Autodesk Fusion 360 part; units mm, degrees
note: some values were not read from the file. Chosen so that the rebuilt part matches the saved one: that a step has no effect.
(part 6 of 7)
  spline S243 degree 3 poles (23.9288, 79.9512) (23.18, 79.2024) (22.4312, 78.4536) (21.6597, 77.6822) knots 0 0 0 0 1 1 1 1
  spline S244 degree 3 poles (21.6597, 77.6822) (21.5445, 77.7398) (21.4293, 77.7974) (21.3106, 77.8567) knots 0 0 0 0 1 1 1 1
  spline S245 degree 3 poles (21.3106, 77.8567) (22.7527, 79.5314) (22.7527, 79.5314) (23.5797, 80.1258) knots 0 0 0 0 1 1 1 1
  spline S246 degree 3 poles (-14.8203, 67.384) (-14.7051, 67.3264) (-14.5899, 67.2688) (-14.4712, 67.2094) knots 0 0 0 0 1 1 1 1
  spline S247 degree 3 poles (-14.4712, 67.2094) (-15.0472, 66.6334) (-15.6232, 66.0574) (-16.2166, 65.464) knots 0 0 0 0 1 1 1 1
  spline S248 degree 3 poles (-16.2166, 65.464) (-16.3318, 65.5216) (-16.447, 65.5792) (-16.5657, 65.6385) knots 0 0 0 0 1 1 1 1
  spline S249 degree 3 poles (-16.5657, 65.6385) (-16.5081, 65.7537) (-16.4505, 65.8689) (-16.3912, 65.9876) knots 0 0 0 0 1 1 1 1
  spline S250 degree 3 poles (-16.3912, 65.9876) (-16.276, 65.9876) (-16.1608, 65.9876) (-16.0421, 65.9876) knots 0 0 0 0 1 1 1 1
  spline S251 degree 3 poles (-16.0421, 65.9876) (-16.0421, 66.1028) (-16.0421, 66.218) (-16.0421, 66.3367) knots 0 0 0 0 1 1 1 1
  spline S252 degree 3 poles (-16.0421, 66.3367) (-15.9269, 66.3367) (-15.8117, 66.3367) (-15.693, 66.3367) knots 0 0 0 0 1 1 1 1
  spline S253 degree 3 poles (-15.693, 66.3367) (-15.693, 66.4519) (-15.693, 66.5671) (-15.693, 66.6858) knots 0 0 0 0 1 1 1 1
  spline S254 degree 3 poles (-15.693, 66.6858) (-15.5778, 66.6858) (-15.4626, 66.6858) (-15.3439, 66.6858) knots 0 0 0 0 1 1 1 1
  spline S255 degree 3 poles (-15.3439, 66.6858) (-15.2863, 66.8586) (-15.2287, 67.0314) (-15.1694, 67.2094) knots 0 0 0 0 1 1 1 1
  spline S256 degree 3 poles (-15.1694, 67.2094) (-15.0542, 67.267) (-14.939, 67.3246) (-14.8203, 67.384) knots 0 0 0 0 1 1 1 1
  spline S257 degree 3 poles (-17.2639, 64.7658) (-17.0911, 64.6506) (-16.9183, 64.5354) (-16.7403, 64.4167) knots 0 0 0 0 1 1 1 1
  spline S258 degree 3 poles (-16.7403, 64.4167) (-16.9357, 64.2411) (-17.1323, 64.0668) (-17.3293, 63.8931) knots 0 0 0 0 1 1 1 1
  spline S259 degree 3 poles (-17.3293, 63.8931) (-17.4387, 63.7959) (-17.548, 63.6987) (-17.6607, 63.5985) knots 0 0 0 0 1 1 1 1
  spline S260 degree 3 poles (-17.6607, 63.5985) (-17.9621, 63.3694) (-17.9621, 63.3694) (-18.3112, 63.3694) knots 0 0 0 0 1 1 1 1
  spline S261 degree 3 poles (-18.3112, 63.3694) (-18.3112, 63.4846) (-18.3112, 63.5998) (-18.3112, 63.7185) knots 0 0 0 0 1 1 1 1
  spline S262 degree 3 poles (-18.3112, 63.7185) (-18.196, 63.7185) (-18.0808, 63.7185) (-17.9621, 63.7185) knots 0 0 0 0 1 1 1 1
  spline S263 degree 3 poles (-17.9621, 63.7185) (-17.9621, 63.8337) (-17.9621, 63.9489) (-17.9621, 64.0676) knots 0 0 0 0 1 1 1 1
  spline S264 degree 3 poles (-17.9621, 64.0676) (-17.8469, 64.0676) (-17.7317, 64.0676) (-17.613, 64.0676) knots 0 0 0 0 1 1 1 1
  spline S265 degree 3 poles (-17.613, 64.0676) (-17.4978, 64.298) (-17.3826, 64.5284) (-17.2639, 64.7658) knots 0 0 0 0 1 1 1 1
sketch "Sketch101" plane through (71.6406, 0, 0) normal (-1, 0, 0) x (0, -1, 0)
  line L0 (57.3648, 64.7338) -> (57.3648, 39.3343)
  line L1 (54.3648, 39.3343) -> (54.3648, 64.7338)
  line L2 (57.3648, 39.3343) -> (54.3648, 39.3343)
  line L3 (54.3648, 39.3343) -> (54.3648, 19.7124)
  line L4 (54.3648, 19.7124) -> (57.3648, 19.7124)
  line L5 (57.3648, 19.7124) -> (57.3648, 39.3343)
  line L6 (57.3648, 39.3343) -> (54.3648, 39.3343)
  line L7 (54.3648, 39.3343) -> (54.3648, 59.6271)
  line L8 (54.3648, 59.6271) -> (57.3648, 59.6271)
  line L9 (57.3648, 59.6271) -> (57.3648, 39.3343)
  constraint horizontal L2
  constraint vertical L3
  constraint horizontal L4
  constraint vertical L5
  constraint coincident L0.end L2.start
  constraint horizontal L6
  constraint vertical L7
  constraint horizontal L8
  constraint vertical L9
  constraint coincident L1 L7.end
extrude "Extrude4" cut sketch "Sketch101" along normal blind 172 and the other way blind 2 bodies 2 in component "Component"
sketch "Sketch102" plane through (0, -58.3648, 0) normal (0, -1, 0) x (1, 0, 0)
  line L0 (76.6406, 106.1458) -> (-103.3594, 106.1458)
  line L1 (-103.3594, 106.1458) -> (-103.3594, 16.8343)
  line L2 (-103.3594, 16.8343) -> (-98.3594, 16.8343)
  line L3 (-98.3594, 16.8343) -> (-98.3594, 39.3343)
  line L4 (-98.3594, 39.3343) -> (-23.3594, 39.3343)
  line L5 (-23.3594, 39.3343) -> (-23.3594, 75)
  line L6 (-23.3594, 75) -> (-3.3594, 75)
  line L7 (-3.3594, 75) -> (-3.3594, 39.3343)
  line L8 (-3.3594, 39.3343) -> (71.6406, 39.3343)
  line L9 (71.6406, 39.3343) -> (71.6406, 16.8343)
  line L10 (71.6406, 16.8343) -> (76.6406, 16.8343)
  line L11 (76.6406, 16.8343) -> (76.6406, 106.1458)
sketch "Sketch103" plane through (0, -58.3648, 0) normal (0, -1, 0) x (1, 0, 0)
  line L0 (-3.3594, 39.3343) -> (-3.3594, 86.8343)
  line L1 (-23.3594, 75) -> (-3.3594, 75)
  line L2 (-23.3594, 39.3343) -> (-23.3594, 75)
  line L3 (-98.3594, 39.3343) -> (-23.3594, 39.3343)
  line L4 (-3.3594, 39.3343) -> (71.6406, 39.3343)
  line L5 (71.6406, 39.3343) -> (71.6406, 16.8343)
  line L6 (76.6406, 16.8343) -> (76.6406, 111.8343)
  line L7 (71.6406, 19.7124) -> (-98.3594, 19.7124)
  line L8 (-98.3594, 16.8343) -> (-98.3594, 39.3343)
  line L9 (-103.3594, 111.8343) -> (-103.3594, 16.8343)
  line L10 (74.0853, 19.7124) -> (-99.6129, 19.7124)
  line L11 (-99.6129, 19.7124) -> (-99.6129, 81.8546)
  line L12 (-99.6129, 81.8546) -> (74.0853, 81.8546)
  line L13 (74.0853, 81.8546) -> (74.0853, 19.7124)
  constraint horizontal L10
  constraint vertical L11
  constraint horizontal L12
  constraint vertical L13
extrude "Extrude32" add sketch "Sketch103" along normal blind 2.5 separate body makes body 3
move_body "Move18" bodies 3 to x (1, 0, 0) y (0, 1, 0) z (0, 0, 1) at (0, -47, 0)
move_body "Move19" bodies 3 to x (1, 0, 0) y (0, 1, 0) z (0, 0, 1) at (0, 50, 0)
sketch "Sketch104" plane through (0, -57.8648, 0) normal (0, -1, 0) x (1, 0, 0)
  line L0 (74.0853, 81.8546) -> (-99.6129, 81.8546)
  line L1 (-99.6129, 81.8546) -> (-99.6129, 19.7124)
  line L2 (-99.6129, 19.7124) -> (74.0853, 19.7124)
  line L3 (74.0853, 19.7124) -> (74.0853, 81.8546)
  line L4 (-8, 43) -> (-19, 43)
  line L5 (-19, 43) -> (-19, 49)
  line L6 (-19, 49) -> (-8, 49)
  line L7 (-8, 49) -> (-8, 43)
  constraint horizontal L4
  constraint vertical L5
  constraint horizontal L6
  constraint vertical L7
extrude "Extrude33" cut sketch "Sketch104" against normal blind 11 contours L4 L5 L6 L7 bodies 3
move_body "Move20" bodies 3 to x (1, 0, 0) y (0, 1, 0) z (0, 0, 1) at (0, -60, 0)
sketch "Sketch105" plane through (0, 0, 0) normal (0, 0, 1) x (1, 0, 0)
sketch "Sketch106" plane through (0, 0, 0) normal (0, 0, 1) x (1, 0, 0)
  line L0 (10, -170) -> (-1, -170)
  line L1 (-1, -170) -> (-1, -162.5)
  line L2 (-1, -162.5) -> (10, -162.5)
  line L3 (10, -162.5) -> (10, -170)
  line L4 (-1, -162.5) -> (2, -162.5)
  line L5 (2, -162.5) -> (2, -158)
  line L6 (2, -158) -> (-1, -158)
  line L7 (-1, -158) -> (-1, -162.5)
  line L8 (10, -162.5) -> (7, -162.5)
  line L9 (7, -162.5) -> (7, -158)
  line L10 (7, -158) -> (10, -158)
  line L11 (10, -158) -> (10, -162.5)
  line L12 (-1, -158) -> (-1, -159.85)
  line L13 (-1, -159.85) -> (-2.25, -159.85)
  line L14 (-2.25, -159.85) -> (-1, -158)
  line L15 (10, -158) -> (10, -159.85)
  line L16 (10, -159.85) -> (11.25, -159.85)
  line L17 (11.25, -159.85) -> (10, -158)
  line L18 (10, -170) -> (11.25, -170)
  line L19 (11.25, -170) -> (11.25, -162.5)
  line L20 (11.25, -162.5) -> (10, -162.5)
  line L21 (10, -162.5) -> (10, -170)
  line L22 (-1, -170) -> (-2.25, -170)
  line L23 (-2.25, -170) -> (-2.25, -162.5)
  line L24 (-2.25, -162.5) -> (-1, -162.5)
  line L25 (-1, -162.5) -> (-1, -170)
  dimension "d167" = 11
  dimension "d168" = 7.5
  dimension "d169" = 4.5
  dimension "d170" = 1.85
  dimension "d171" = 1.25
  dimension "d172" = 1.85
  dimension "d173" = 1.25
  dimension "d174" = 1.25
  dimension "d175" = 1.25
  constraint horizontal L0
  constraint vertical L1
  constraint horizontal L2
  constraint vertical L3
  constraint horizontal L4
  constraint vertical L5
  constraint horizontal L6
  constraint vertical L7
  constraint horizontal L8
  constraint vertical L9
  constraint horizontal L10
  constraint vertical L11
  constraint coincident L7 L12.end
  constraint perpendicular L12 L13
  constraint coincident L11 L15.end
  constraint perpendicular L11 L16
  constraint horizontal L18
  constraint vertical L19
  constraint horizontal L20
  constraint vertical L21
  constraint horizontal L22
  constraint vertical L23
  constraint horizontal L24
  constraint vertical L25
  measures "d167" distance of L0.start L0.end
  measures "d168" distance of L0.start L2.end
  measures "d169" distance of L1.end L6.end
  measures "d170" distance of L6.end L12.end
  measures "d171" distance of L12.end L13.end
  measures "d172" distance of L10.end L15.end
  measures "d173" distance of L15.end L16.end
  measures "d174" distance of L0.start L18.end
  measures "d175" distance of L0.end L22.end
extrude "Extrude34" add sketch "Sketch106" along normal blind 6 separate body makes body 4
fillet "Fillet4" radius 6 tangency weight 1.3685 1 edges at (4.5, -170, 6) on bodies 4
sketch "Sketch59" plane through (-89.5415, 0, 0) normal (-1, 0, 0) x (0, -1, 0)
sketch "Sketch60" plane through (0, 0, 0) normal (1, 0, 0) x (0, 1, 0)
sketch "Sketch107" plane through (0, 66.6352, 0) normal (0, 1, 0) x (-1, 0, 0)
  line L0 (103.3594, 140.242) -> (-76.6406, 140.242)
  line L1 (-76.6406, 140.242) -> (-76.6406, 16.8343)
  line L2 (-76.6406, 16.8343) -> (103.3594, 16.8343)
  line L3 (103.3594, 16.8343) -> (103.3594, 140.242)
  spline S0 degree 3 poles (-45.7064, 96.8261) (-45.5481, 96.8681) (-45.3897, 96.9101) (-45.2266, 96.9534) knots 0 0 0 0 1 1 1 1
  spline S1 degree 3 poles (-45.2266, 96.9534) (-42.4795, 97.6788) (-39.7486, 98.2533) (-36.9248, 98.5683) knots 0 0 0 0 1 1 1 1
  spline S2 degree 3 poles (-36.9248, 98.5683) (-36.7802, 98.5846) (-36.7802, 98.5846) (-36.6326, 98.6012) knots 0 0 0 0 1 1 1 1
  spline S3 degree 3 poles (-36.6326, 98.6012) (-25.791, 99.8038) (-14.8744, 98.8757) (-3.0729, 96.8273) knots 0 0 0 0 1 1 1 1
  spline S4 degree 3 poles (-3.0729, 96.8273) (8.3921, 94.7476) (19.8407, 95.0185) (31.1023, 98.0497) knots 0 0 0 0 1 1 1 1
  spline S5 degree 3 poles (31.1023, 98.0497) (31.2954, 98.1015) (31.2954, 98.1015) (31.4923, 98.1544) knots 0 0 0 0 1 1 1 1
  spline S6 degree 3 poles (31.4923, 98.1544) (33.7602, 98.766) (35.989, 99.441) (38.1951, 100.2513) knots 0 0 0 0 1 1 1 1
  spline S7 degree 3 poles (38.1951, 100.2513) (38.2806, 100.2826) (38.3662, 100.3138) (38.4543, 100.3461) knots 0 0 0 0 1 1 1 1
  spline S8 degree 3 poles (38.4543, 100.3461) (48.019, 103.8522) (56.949, 108.978) (65.0365, 115.1519) knots 0 0 0 0 1 1 1 1
  spline S9 degree 3 poles (65.0365, 115.1519) (65.1117, 115.2093) (65.1868, 115.2666) (65.2643, 115.3258) knots 0 0 0 0 1 1 1 1
  spline S10 degree 3 poles (65.2643, 115.3258) (69.065, 118.2344) (72.9424, 121.3668) (76.1266, 124.9512) knots 0 0 0 0 1 1 1 1
  spline S11 degree 3 poles (76.1266, 124.9512) (76.5375, 125.3995) (76.5375, 125.3995) (76.9194, 125.4556) knots 0 0 0 0 1 1 1 1
  spline S12 degree 3 poles (76.9194, 125.4556) (77.0345, 125.4372) (77.0345, 125.4372) (77.152, 125.4185) knots 0 0 0 0 1 1 1 1
  spline S13 degree 3 poles (77.152, 125.4185) (77.4126, 125.0218) (77.4195, 124.9501) (77.3533, 124.4429) knots 0 0 0 0 1 1 1 1
  spline S14 degree 3 poles (77.3533, 124.4429) (77.3089, 124.2369) (77.2625, 124.0312) (77.2147, 123.8259) knots 0 0 0 0 1 1 1 1
  spline S15 degree 3 poles (77.2147, 123.8259) (77.1901, 123.7141) (77.1655, 123.6022) (77.1402, 123.4869) knots 0 0 0 0 1 1 1 1
  spline S16 degree 3 poles (77.1402, 123.4869) (77.0586, 123.1177) (76.9746, 122.749) (76.8906, 122.3803) knots 0 0 0 0 1 1 1 1
  spline S17 degree 3 poles (76.8906, 122.3803) (76.8333, 122.1227) (76.7762, 121.865) (76.7192, 121.6073) knots 0 0 0 0 1 1 1 1
  spline S18 degree 3 poles (76.7192, 121.6073) (76.6019, 121.0775) (76.4837, 120.5479) (76.3648, 120.0184) knots 0 0 0 0 1 1 1 1
  spline S19 degree 3 poles (76.3648, 120.0184) (76.2043, 119.3015) (76.0477, 118.5839) (75.8931, 117.8657) knots 0 0 0 0 1 1 1 1
  spline S20 degree 3 poles (75.8931, 117.8657) (75.8697, 117.7573) (75.8464, 117.6488) (75.8223, 117.5371) knots 0 0 0 0 1 1 1 1
  spline S21 degree 3 poles (75.8223, 117.5371) (75.7761, 117.3223) (75.7299, 117.1075) (75.6837, 116.8927) knots 0 0 0 0 1 1 1 1
  spline S22 degree 3 poles (75.6837, 116.8927) (75.4001, 115.5741) (75.1139, 114.2561) (74.8196, 112.9399) knots 0 0 0 0 1 1 1 1
  spline S23 degree 3 poles (74.8196, 112.9399) (74.7781, 112.7534) (74.7365, 112.5669) (74.695, 112.3805) knots 0 0 0 0 1 1 1 1
  spline S24 degree 3 poles (74.695, 112.3805) (74.6179, 112.035) (74.5401, 111.6897) (74.4619, 111.3445) knots 0 0 0 0 1 1 1 1
  spline S25 degree 3 poles (74.4619, 111.3445) (74.4282, 111.1936) (74.3945, 111.0428) (74.3598, 110.8874) knots 0 0 0 0 1 1 1 1
  spline S26 degree 3 poles (74.3598, 110.8874) (74.3301, 110.7558) (74.3004, 110.6243) (74.2697, 110.4887) knots 0 0 0 0 1 1 1 1
  spline S27 degree 3 poles (74.2697, 110.4887) (74.1941, 110.1853) (74.1941, 110.1853) (74.2842, 109.9213) knots 0 0 0 0 1 1 1 1
  spline S28 degree 3 poles (74.2842, 109.9213) (76.0956, 110.302) (77.8875, 110.7306) (79.6733, 111.2173) knots 0 0 0 0 1 1 1 1
  spline S29 degree 3 poles (79.6733, 111.2173) (80.0659, 111.3243) (80.4588, 111.4304) (80.8516, 111.5364) knots 0 0 0 0 1 1 1 1
  spline S30 degree 3 poles (80.8516, 111.5364) (81.6816, 111.7603) (82.5112, 111.9853) (83.3409, 112.2104) knots 0 0 0 0 1 1 1 1
  spline S31 degree 3 poles (83.3409, 112.2104) (84.3124, 112.474) (85.284, 112.7371) (86.2558, 112.9991) knots 0 0 0 0 1 1 1 1
  spline S32 degree 3 poles (86.2558, 112.9991) (86.6428, 113.1037) (87.0296, 113.2091) (87.4163, 113.3145) knots 0 0 0 0 1 1 1 1
  spline S33 degree 3 poles (87.4163, 113.3145) (87.6511, 113.3779) (87.8859, 113.4412) (88.1207, 113.5046) knots 0 0 0 0 1 1 1 1
  spline S34 degree 3 poles (88.1207, 113.5046) (88.228, 113.5341) (88.3354, 113.5635) (88.446, 113.5939) knots 0 0 0 0 1 1 1 1
  spline S35 degree 3 poles (88.446, 113.5939) (89.1834, 113.7916) (89.1834, 113.7916) (89.5079, 113.7252) knots 0 0 0 0 1 1 1 1
  spline S36 degree 3 poles (89.5079, 113.7252) (89.5844, 113.1789) (89.5219, 112.9091) (89.2263, 112.4463) knots 0 0 0 0 1 1 1 1
  spline S37 degree 3 poles (89.2263, 112.4463) (89.156, 112.3347) (89.0857, 112.2231) (89.0134, 112.1081) knots 0 0 0 0 1 1 1 1
  spline S38 degree 3 poles (89.0134, 112.1081) (88.9387, 111.9931) (88.864, 111.8782) (88.787, 111.7598) knots 0 0 0 0 1 1 1 1
  spline S39 degree 3 poles (88.787, 111.7598) (88.6798, 111.5902) (88.6798, 111.5902) (88.5704, 111.4173) knots 0 0 0 0 1 1 1 1
  spline S40 degree 3 poles (88.5704, 111.4173) (87.8976, 110.3582) (87.1937, 109.32) (86.483, 108.2861) knots 0 0 0 0 1 1 1 1
  spline S41 degree 3 poles (86.483, 108.2861) (86.049, 107.6537) (85.6171, 107.0201) (85.188, 106.3844) knots 0 0 0 0 1 1 1 1
  spline S42 degree 3 poles (85.188, 106.3844) (84.1912, 104.9075) (83.192, 103.4375) (82.1157, 102.017) knots 0 0 0 0 1 1 1 1
  spline S43 degree 3 poles (82.1157, 102.017) (81.6377, 101.3842) (81.1782, 100.7395) (80.7206, 100.0918) knots 0 0 0 0 1 1 1 1
  spline S44 degree 3 poles (80.7206, 100.0918) (80.0586, 99.1578) (79.3691, 98.2516) (78.6566, 97.3557) knots 0 0 0 0 1 1 1 1
  spline S45 degree 3 poles (78.6566, 97.3557) (78.2349, 96.8249) (77.8215, 96.288) (77.4084, 95.7505) knots 0 0 0 0 1 1 1 1
  spline S46 degree 3 poles (77.4084, 95.7505) (76.5588, 94.6451) (75.7018, 93.5492) (74.8053, 92.4814) knots 0 0 0 0 1 1 1 1
  spline S47 degree 3 poles (74.8053, 92.4814) (74.5969, 92.2324) (74.39, 91.9821) (74.1832, 91.7317) knots 0 0 0 0 1 1 1 1
  spline S48 degree 3 poles (74.1832, 91.7317) (67.0705, 83.1524) (59.1895, 75.0046) (40.5169, 63.8451) knots 0 0 0 0 1 1 1 1
  spline S49 degree 3 poles (40.5169, 63.8451) (40.3871, 63.7934) (40.2573, 63.7418) (40.1236, 63.6886) knots 0 0 0 0 1 1 1 1
  spline S50 degree 3 poles (40.1236, 63.6886) (28.4595, 59.163) (14.8221, 57.7208) (-16.1582, 57.4264) knots 0 0 0 0 1 1 1 1
  spline S51 degree 3 poles (-16.1582, 57.4264) (-32.9463, 58.0691) (-32.9463, 58.0691) (-50.0558, 56.645) knots 0 0 0 0 1 1 1 1
  spline S52 degree 3 poles (-50.0558, 56.645) (-50.1821, 56.6269) (-50.3084, 56.6088) (-50.4385, 56.5901) knots 0 0 0 0 1 1 1 1
  spline S53 degree 3 poles (-50.4385, 56.5901) (-54.3089, 56.0263) (-58.132, 54.9004) (-61.7438, 53.4135) knots 0 0 0 0 1 1 1 1
  spline S54 degree 3 poles (-61.7438, 53.4135) (-62.1127, 53.2747) (-62.4824, 53.1713) (-62.8645, 53.0753) knots 0 0 0 0 1 1 1 1
  spline S55 degree 3 poles (-62.8645, 53.0753) (-62.2573, 46.7418) (-61.3762, 40.5103) (-59.846, 34.3289) knots 0 0 0 0 1 1 1 1
  spline S56 degree 3 poles (-59.846, 34.3289) (-59.778, 34.0527) (-59.71, 33.7766) (-59.642, 33.5004) knots 0 0 0 0 1 1 1 1
  spline S57 degree 3 poles (-59.642, 33.5004) (-59.4776, 32.8323) (-59.3124, 32.1643) (-59.1472, 31.4964) knots 0 0 0 0 1 1 1 1
  spline S58 degree 3 poles (-59.1472, 31.4964) (-60.7154, 31.0762) (-62.2835, 30.656) (-63.8992, 30.2231) knots 0 0 0 0 1 1 1 1
  spline S59 degree 3 poles (-63.8992, 30.2231) (-67.1692, 41.0011) (-67.0232, 53.7045) (-63.94, 78.6656) knots 0 0 0 0 1 1 1 1
  spline S60 degree 3 poles (-63.94, 78.6656) (-63.9131, 78.8142) (-63.8861, 78.9628) (-63.8583, 79.1159) knots 0 0 0 0 1 1 1 1
  spline S61 degree 3 poles (-63.8583, 79.1159) (-63.665, 80.175) (-63.4644, 81.2325) (-63.2592, 82.2893) knots 0 0 0 0 1 1 1 1
  spline S62 degree 3 poles (-63.2592, 82.2893) (-63.2291, 82.4451) (-63.1989, 82.6008) (-63.1679, 82.7613) knots 0 0 0 0 1 1 1 1
  spline S63 degree 3 poles (-63.1679, 82.7613) (-61.8055, 89.7543) (-61.8055, 89.7543) (-61.1055, 90.6265) knots 0 0 0 0 1 1 1 1
  spline S64 degree 3 poles (-61.1055, 90.6265) (-60.7716, 90.8303) (-60.4678, 90.9184) (-60.0835, 90.9864) knots 0 0 0 0 1 1 1 1
  spline S65 degree 3 poles (-60.0835, 90.9864) (-59.7353, 90.7854) (-59.6641, 90.6676) (-59.4917, 90.3191) knots 0 0 0 0 1 1 1 1
  spline S66 degree 3 poles (-59.4917, 90.3191) (-59.4098, 90.3895) (-59.3279, 90.4599) (-59.2435, 90.5324) knots 0 0 0 0 1 1 1 1
  spline S67 degree 3 poles (-59.2435, 90.5324) (-55.3519, 93.7416) (-50.5292, 95.5611) (-45.7064, 96.8261) knots 0 0 0 0 1 1 1 1
  spline S68 degree 3 poles (-48.2512, 87.4119) (-47.2839, 87.3215) (-46.6105, 86.7927) (-45.9714, 86.0957) knots 0 0 0 0 1 1 1 1
  spline S69 degree 3 poles (-45.9714, 86.0957) (-45.6421, 85.688) (-45.3536, 85.2668) (-45.0791, 84.8206) knots 0 0 0 0 1 1 1 1
  spline S70 degree 3 poles (-45.0791, 84.8206) (-45.024, 84.7314) (-44.9689, 84.6422) (-44.9121, 84.5503) knots 0 0 0 0 1 1 1 1
  spline S71 degree 3 poles (-44.9121, 84.5503) (-44.1771, 83.2187) (-43.8013, 81.5801) (-43.8059, 80.0686) knots 0 0 0 0 1 1 1 1
  spline S72 degree 3 poles (-43.8059, 80.0686) (-43.7534, 79.8533) (-43.697, 79.6389) (-43.6338, 79.4265) knots 0 0 0 0 1 1 1 1
  spline S73 degree 3 poles (-43.6338, 79.4265) (-42.0204, 79.1867) (-40.4101, 78.9482) (-38.7854, 78.7985) knots 0 0 0 0 1 1 1 1
  spline S74 degree 3 poles (-38.7854, 78.7985) (-38.7949, 78.8939) (-38.8045, 78.9892) (-38.8144, 79.0875) knots 0 0 0 0 1 1 1 1
  spline S75 degree 3 poles (-38.8144, 79.0875) (-38.8299, 79.4995) (-38.7836, 79.8578) (-38.714, 80.264) knots 0 0 0 0 1 1 1 1
  spline S76 degree 3 poles (-38.714, 80.264) (-38.688, 80.417) (-38.6619, 80.57) (-38.635, 80.7276) knots 0 0 0 0 1 1 1 1
  spline S77 degree 3 poles (-38.635, 80.7276) (-38.6063, 80.8899) (-38.5775, 81.0522) (-38.5479, 81.2194) knots 0 0 0 0 1 1 1 1
  spline S78 degree 3 poles (-38.5479, 81.2194) (-38.5186, 81.3862) (-38.4893, 81.553) (-38.4591, 81.7249) knots 0 0 0 0 1 1 1 1
  spline S79 degree 3 poles (-38.4591, 81.7249) (-38.276, 82.7484) (-38.0824, 83.769) (-37.86, 84.7848) knots 0 0 0 0 1 1 1 1
  spline S80 degree 3 poles (-37.86, 84.7848) (-37.837, 84.8937) (-37.8139, 85.0025) (-37.7901, 85.1147) knots 0 0 0 0 1 1 1 1
  spline S81 degree 3 poles (-37.7901, 85.1147) (-37.5744, 86.0609) (-37.2674, 87.0489) (-36.4835, 87.6744) knots 0 0 0 0 1 1 1 1
  spline S82 degree 3 poles (-36.4835, 87.6744) (-35.8146, 87.9652) (-35.173, 88.1221) (-34.4492, 88.013) knots 0 0 0 0 1 1 1 1
  spline S83 degree 3 poles (-34.4492, 88.013) (-33.7177, 87.6026) (-33.1504, 87.1937) (-32.9061, 86.3596) knots 0 0 0 0 1 1 1 1
  spline S84 degree 3 poles (-32.9061, 86.3596) (-32.6181, 85.1833) (-32.6635, 83.9595) (-32.6534, 82.7558) knots 0 0 0 0 1 1 1 1
  spline S85 degree 3 poles (-32.6534, 82.7558) (-32.6518, 82.6241) (-32.6501, 82.4924) (-32.6484, 82.3567) knots 0 0 0 0 1 1 1 1
  spline S86 degree 3 poles (-32.6484, 82.3567) (-32.6146, 79.6527) (-32.6761, 76.9545) (-32.7882, 74.253) knots 0 0 0 0 1 1 1 1
  spline S87 degree 3 poles (-32.7882, 74.253) (-32.8012, 73.9352) (-32.8133, 73.6174) (-32.8251, 73.2995) knots 0 0 0 0 1 1 1 1
  spline S88 degree 3 poles (-32.8251, 73.2995) (-32.8438, 72.8023) (-32.8641, 72.3051) (-32.886, 71.808) knots 0 0 0 0 1 1 1 1
  spline S89 degree 3 poles (-32.886, 71.808) (-32.8975, 71.5439) (-32.9079, 71.2798) (-32.9184, 71.0157) knots 0 0 0 0 1 1 1 1
  spline S90 degree 3 poles (-32.9184, 71.0157) (-33.0049, 69.2409) (-33.1993, 67.4218) (-34.4428, 66.0593) knots 0 0 0 0 1 1 1 1
  spline S91 degree 3 poles (-34.4428, 66.0593) (-35.0109, 65.5526) (-35.6375, 65.3103) (-36.3967, 65.2604) knots 0 0 0 0 1 1 1 1
  spline S92 degree 3 poles (-36.3967, 65.2604) (-36.9978, 65.4856) (-37.2892, 65.7801) (-37.6399, 66.3038) knots 0 0 0 0 1 1 1 1
  spline S93 degree 3 poles (-37.6399, 66.3038) (-38.0544, 67.3349) (-38.0845, 68.4101) (-38.111, 69.507) knots 0 0 0 0 1 1 1 1
  spline S94 degree 3 poles (-38.111, 69.507) (-38.1217, 69.831) (-38.1327, 70.155) (-38.144, 70.479) knots 0 0 0 0 1 1 1 1
  spline S95 degree 3 poles (-38.144, 70.479) (-38.1492, 70.6346) (-38.1543, 70.7903) (-38.1597, 70.9506) knots 0 0 0 0 1 1 1 1
  spline S96 degree 3 poles (-38.1597, 70.9506) (-38.1938, 71.8188) (-38.2651, 72.6835) (-38.3423, 73.5488) knots 0 0 0 0 1 1 1 1
  spline S97 degree 3 poles (-38.3423, 73.5488) (-38.416, 73.549) (-38.4896, 73.5492) (-38.5655, 73.5494) knots 0 0 0 0 1 1 1 1
  spline S98 degree 3 poles (-38.5655, 73.5494) (-39.7226, 73.5671) (-40.8652, 73.7004) (-42.0137, 73.8297) knots 0 0 0 0 1 1 1 1
  spline S99 degree 3 poles (-42.0137, 73.8297) (-42.2191, 73.8524) (-42.4245, 73.8751) (-42.6299, 73.8977) knots 0 0 0 0 1 1 1 1
  spline S100 degree 3 poles (-42.6299, 73.8977) (-43.128, 73.9527) (-43.6261, 74.0083) (-44.1241, 74.0643) knots 0 0 0 0 1 1 1 1
  spline S101 degree 3 poles (-44.1241, 74.0643) (-44.1289, 73.9442) (-44.1337, 73.8241) (-44.1387, 73.7003) knots 0 0 0 0 1 1 1 1
  spline S102 degree 3 poles (-44.1387, 73.7003) (-44.1936, 72.9724) (-44.3564, 72.2721) (-44.512, 71.5599) knots 0 0 0 0 1 1 1 1
  spline S103 degree 3 poles (-44.512, 71.5599) (-44.5686, 71.2988) (-44.6228, 71.0371) (-44.677, 70.7755) knots 0 0 0 0 1 1 1 1
  spline S104 degree 3 poles (-44.677, 70.7755) (-44.9743, 69.4058) (-45.3183, 68.0168) (-46.3334, 66.9941) knots 0 0 0 0 1 1 1 1
  spline S105 degree 3 poles (-46.3334, 66.9941) (-46.432, 66.8923) (-46.5305, 66.7905) (-46.632, 66.6856) knots 0 0 0 0 1 1 1 1
  spline S106 degree 3 poles (-46.632, 66.6856) (-47.2185, 66.1416) (-47.8826, 65.9502) (-48.6622, 65.8281) knots 0 0 0 0 1 1 1 1
  spline S107 degree 3 poles (-48.6622, 65.8281) (-49.2058, 65.9712) (-49.5103, 66.1644) (-49.8365, 66.6147) knots 0 0 0 0 1 1 1 1
  spline S108 degree 3 poles (-49.8365, 66.6147) (-50.4305, 68.1882) (-50.5246, 69.623) (-50.3988, 71.2818) knots 0 0 0 0 1 1 1 1
  spline S109 degree 3 poles (-50.3988, 71.2818) (-50.1218, 75.1545) (-50.1421, 78.9743) (-50.4328, 82.8449) knots 0 0 0 0 1 1 1 1
  spline S110 degree 3 poles (-50.4328, 82.8449) (-50.6339, 85.6223) (-50.6339, 85.6223) (-49.977, 86.4677) knots 0 0 0 0 1 1 1 1
  spline S111 degree 3 poles (-49.977, 86.4677) (-49.9171, 86.5476) (-49.8573, 86.6276) (-49.7956, 86.7099) knots 0 0 0 0 1 1 1 1
  spline S112 degree 3 poles (-49.7956, 86.7099) (-49.3755, 87.2034) (-48.8822, 87.3316) (-48.2512, 87.4119) knots 0 0 0 0 1 1 1 1
  spline S113 degree 3 poles (-60.0835, 90.9864) (-59.9223, 90.8933) (-59.9223, 90.8933) (-59.7578, 90.7984) knots 0 0 0 0 1 1 1 1
  spline S114 degree 3 poles (-59.7578, 90.7984) (-59.6284, 90.1547) (-59.6564, 89.6237) (-59.7823, 88.9835) knots 0 0 0 0 1 1 1 1
  spline S115 degree 3 poles (-59.7823, 88.9835) (-59.8155, 88.8087) (-59.8487, 88.6338) (-59.8818, 88.4589) knots 0 0 0 0 1 1 1 1
  spline S116 degree 3 poles (-59.8818, 88.4589) (-59.8999, 88.3664) (-59.918, 88.2739) (-59.9366, 88.1786) knots 0 0 0 0 1 1 1 1
  spline S117 degree 3 poles (-59.9366, 88.1786) (-61.1903, 81.7212) (-61.9509, 75.1546) (-62.5143, 68.604) knots 0 0 0 0 1 1 1 1
  spline S118 degree 3 poles (-62.5143, 68.604) (-62.5403, 68.3024) (-62.5667, 68.001) (-62.5932, 67.6995) knots 0 0 0 0 1 1 1 1
  spline S119 degree 3 poles (-62.5932, 67.6995) (-63.012, 62.906) (-63.2982, 58.0622) (-62.8373, 53.2629) knots 0 0 0 0 1 1 1 1
  spline S120 degree 3 poles (-62.8373, 53.2629) (-62.7985, 52.8482) (-62.7622, 52.4335) (-62.7269, 52.0185) knots 0 0 0 0 1 1 1 1
  spline S121 degree 3 poles (-62.7269, 52.0185) (-62.2171, 46.0375) (-61.2886, 40.1566) (-59.846, 34.3289) knots 0 0 0 0 1 1 1 1
  spline S122 degree 3 poles (-59.846, 34.3289) (-59.778, 34.0527) (-59.71, 33.7766) (-59.642, 33.5004) knots 0 0 0 0 1 1 1 1
  spline S123 degree 3 poles (-59.642, 33.5004) (-59.4776, 32.8323) (-59.3124, 32.1643) (-59.1472, 31.4964) knots 0 0 0 0 1 1 1 1
  spline S124 degree 3 poles (-59.1472, 31.4964) (-60.7154, 31.0762) (-62.2835, 30.656) (-63.8992, 30.2231) knots 0 0 0 0 1 1 1 1
  spline S125 degree 3 poles (-63.8992, 30.2231) (-67.1692, 41.0011) (-67.0232, 53.7045) (-63.94, 78.6656) knots 0 0 0 0 1 1 1 1
  spline S126 degree 3 poles (-63.94, 78.6656) (-63.9131, 78.8142) (-63.8861, 78.9628) (-63.8583, 79.1159) knots 0 0 0 0 1 1 1 1
  spline S127 degree 3 poles (-63.8583, 79.1159) (-63.665, 80.175) (-63.4644, 81.2325) (-63.2592, 82.2893) knots 0 0 0 0 1 1 1 1
  spline S128 degree 3 poles (-63.2592, 82.2893) (-63.2291, 82.4451) (-63.1989, 82.6008) (-63.1679, 82.7613) knots 0 0 0 0 1 1 1 1
  spline S129 degree 3 poles (-63.1679, 82.7613) (-61.8055, 89.7543) (-61.8055, 89.7543) (-61.1055, 90.6265) knots 0 0 0 0 1 1 1 1
  spline S130 degree 3 poles (-61.1055, 90.6265) (-60.7716, 90.8303) (-60.4678, 90.9184) (-60.0835, 90.9864) knots 0 0 0 0 1 1 1 1
  spline S131 degree 3 poles (-21.8651, 89.1136) (-20.6908, 88.715) (-19.8867, 87.8368) (-19.3239, 86.7576) knots 0 0 0 0 1 1 1 1
  spline S132 degree 3 poles (-19.3239, 86.7576) (-16.9734, 81.8605) (-16.4757, 75.9409) (-16.3625, 70.5683) knots 0 0 0 0 1 1 1 1
  spline S133 degree 3 poles (-16.3625, 70.5683) (-16.3598, 70.4405) (-16.3571, 70.3127) (-16.3543, 70.181) knots 0 0 0 0 1 1 1 1
  spline S134 degree 3 poles (-16.3543, 70.181) (-16.3393, 68.545) (-16.5087, 67.1547) (-17.5603, 65.8318) knots 0 0 0 0 1 1 1 1
  spline S135 degree 3 poles (-17.5603, 65.8318) (-18.072, 65.3272) (-18.6716, 65.0325) (-19.3953, 64.9981) knots 0 0 0 0 1 1 1 1
  spline S136 degree 3 poles (-19.3953, 64.9981) (-19.9203, 65.1264) (-20.2664, 65.3255) (-20.5696, 65.7847) knots 0 0 0 0 1 1 1 1
  spline S137 degree 3 poles (-20.5696, 65.7847) (-20.8221, 66.5469) (-20.8732, 67.1817) (-20.8262, 67.9786) knots 0 0 0 0 1 1 1 1
  spline S138 degree 3 poles (-20.8262, 67.9786) (-20.8212, 68.0853) (-20.8162, 68.192) (-20.811, 68.302) knots 0 0 0 0 1 1 1 1
  spline S139 degree 3 poles (-20.811, 68.302) (-20.7948, 68.6391) (-20.7764, 68.9761) (-20.758, 69.3131) knots 0 0 0 0 1 1 1 1
  spline S140 degree 3 poles (-20.758, 69.3131) (-20.7465, 69.5432) (-20.7352, 69.7734) (-20.7241, 70.0035) knots 0 0 0 0 1 1 1 1
  spline S141 degree 3 poles (-20.7241, 70.0035) (-20.6966, 70.5643) (-20.6672, 71.125) (-20.6366, 71.6857) knots 0 0 0 0 1 1 1 1
  spline S142 degree 3 poles (-20.6366, 71.6857) (-20.7837, 71.6554) (-20.9308, 71.625) (-21.0824, 71.5937) knots 0 0 0 0 1 1 1 1
  spline S143 degree 3 poles (-21.0824, 71.5937) (-23.0119, 71.1956) (-23.0119, 71.1956) (-23.9734, 71.0067) knots 0 0 0 0 1 1 1 1
  spline S144 degree 3 poles (-23.9734, 71.0067) (-24.2164, 70.9589) (-24.2164, 70.9589) (-24.4642, 70.9102) knots 0 0 0 0 1 1 1 1
  spline S145 degree 3 poles (-24.4642, 70.9102) (-24.5801, 70.8875) (-24.6959, 70.8648) (-24.8152, 70.8414) knots 0 0 0 0 1 1 1 1
  spline S146 degree 3 poles (-24.8152, 70.8414) (-24.8424, 70.7308) (-24.8695, 70.6203) (-24.8975, 70.5064) knots 0 0 0 0 1 1 1 1
  spline S147 degree 3 poles (-24.8975, 70.5064) (-25.3248, 68.8463) (-25.8405, 67.3953) (-27.0852, 66.181) knots 0 0 0 0 1 1 1 1
  spline S148 degree 3 poles (-27.0852, 66.181) (-27.5079, 65.9563) (-27.8345, 65.9103) (-28.3123, 65.9124) knots 0 0 0 0 1 1 1 1
  spline S149 degree 3 poles (-28.3123, 65.9124) (-28.8844, 66.2427) (-29.155, 66.555) (-29.3745, 67.1796) knots 0 0 0 0 1 1 1 1
  spline S150 degree 3 poles (-29.3745, 67.1796) (-29.4836, 67.7325) (-29.4364, 68.0722) (-29.3134, 68.6209) knots 0 0 0 0 1 1 1 1
  spline S151 degree 3 poles (-29.3134, 68.6209) (-29.2812, 68.7666) (-29.2812, 68.7666) (-29.2485, 68.9153) knots 0 0 0 0 1 1 1 1
  spline S152 degree 3 poles (-29.2485, 68.9153) (-28.9496, 70.242) (-28.6124, 71.5605) (-28.2827, 72.8798) knots 0 0 0 0 1 1 1 1
  spline S153 degree 3 poles (-28.2827, 72.8798) (-27.9632, 74.1588) (-27.6575, 75.4407) (-27.3563, 76.7242) knots 0 0 0 0 1 1 1 1
  spline S154 degree 3 poles (-27.3563, 76.7242) (-27.0922, 77.849) (-26.8196, 78.9716) (-26.5437, 80.0936) knots 0 0 0 0 1 1 1 1
  spline S155 degree 3 poles (-26.5437, 80.0936) (-26.3612, 80.844) (-26.1906, 81.5962) (-26.0303, 82.3517) knots 0 0 0 0 1 1 1 1
  spline S156 degree 3 poles (-26.0303, 82.3517) (-26.0117, 82.4391) (-25.993, 82.5264) (-25.9738, 82.6164) knots 0 0 0 0 1 1 1 1
  spline S157 degree 3 poles (-25.9738, 82.6164) (-25.883, 83.0417) (-25.7936, 83.4671) (-25.7067, 83.8931) knots 0 0 0 0 1 1 1 1
  spline S158 degree 3 poles (-25.7067, 83.8931) (-25.3443, 85.6037) (-24.843, 87.2499) (-23.5784, 88.5083) knots 0 0 0 0 1 1 1 1
  spline S159 degree 3 poles (-23.5784, 88.5083) (-23.0404, 88.8359) (-22.4997, 89.0753) (-21.8651, 89.1136) knots 0 0 0 0 1 1 1 1
  spline S160 degree 3 poles (3.4549, 87.0884) (4.522, 86.7497) (5.3416, 86.0932) (5.9068, 85.13) knots 0 0 0 0 1 1 1 1
  spline S161 degree 3 poles (5.9068, 85.13) (6.0313, 84.7783) (6.1371, 84.4408) (6.2308, 84.0812) knots 0 0 0 0 1 1 1 1
  spline S162 degree 3 poles (6.2308, 84.0812) (6.2582, 83.9778) (6.2856, 83.8745) (6.3139, 83.768) knots 0 0 0 0 1 1 1 1
  spline S163 degree 3 poles (6.3139, 83.768) (6.6867, 82.2839) (6.8686, 80.7622) (7.0701, 79.2474) knots 0 0 0 0 1 1 1 1
  spline S164 degree 3 poles (7.0701, 79.2474) (7.099, 79.0363) (7.1281, 78.8253) (7.1574, 78.6142) knots 0 0 0 0 1 1 1 1
  spline S165 degree 3 poles (7.1574, 78.6142) (7.1771, 78.4728) (7.1967, 78.3313) (7.2169, 78.1855) knots 0 0 0 0 1 1 1 1
  spline S166 degree 3 poles (7.2169, 78.1855) (7.273, 78.303) (7.273, 78.303) (7.3302, 78.4229) knots 0 0 0 0 1 1 1 1
  spline S167 degree 3 poles (7.3302, 78.4229) (7.9064, 79.6144) (8.5482, 80.6858) (9.3322, 81.7537) knots 0 0 0 0 1 1 1 1
  spline S168 degree 3 poles (9.3322, 81.7537) (9.5621, 82.073) (9.7738, 82.3962) (9.9827, 82.7292) knots 0 0 0 0 1 1 1 1
  spline S169 degree 3 poles (9.9827, 82.7292) (10.5648, 83.5982) (11.283, 84.5535) (12.3173, 84.8689) knots 0 0 0 0 1 1 1 1
  spline S170 degree 3 poles (12.3173, 84.8689) (12.9622, 84.9365) (12.9622, 84.9365) (13.333, 84.6421) knots 0 0 0 0 1 1 1 1
  spline S171 degree 3 poles (13.333, 84.6421) (13.78, 83.8277) (13.6923, 82.984) (13.4817, 82.1128) knots 0 0 0 0 1 1 1 1
  spline S172 degree 3 poles (13.4817, 82.1128) (12.8172, 80.0529) (11.7413, 78.0653) (10.6367, 76.2111) knots 0 0 0 0 1 1 1 1
  spline S173 degree 3 poles (10.6367, 76.2111) (10.8545, 75.9616) (11.0765, 75.7193) (11.3066, 75.4808) knots 0 0 0 0 1 1 1 1
  spline S174 degree 3 poles (11.3066, 75.4808) (13.1856, 73.4756) (15.6907, 70.2715) (15.7518, 67.3955) knots 0 0 0 0 1 1 1 1
  spline S175 degree 3 poles (15.7518, 67.3955) (15.7059, 66.6774) (15.5609, 66.0341) (15.0089, 65.5446) knots 0 0 0 0 1 1 1 1
  spline S176 degree 3 poles (15.0089, 65.5446) (14.2673, 65.2091) (13.5854, 65.0209) (12.8016, 65.3059) knots 0 0 0 0 1 1 1 1
  spline S177 degree 3 poles (12.8016, 65.3059) (11.6131, 65.8346) (11.2089, 66.8764) (10.7204, 68.0003) knots 0 0 0 0 1 1 1 1
  spline S178 degree 3 poles (10.7204, 68.0003) (10.5783, 68.3181) (10.4357, 68.6357) (10.2925, 68.9529) knots 0 0 0 0 1 1 1 1
  spline S179 degree 3 poles (10.2925, 68.9529) (10.256, 69.034) (10.2194, 69.115) (10.1818, 69.1985) knots 0 0 0 0 1 1 1 1
  spline S180 degree 3 poles (10.1818, 69.1985) (9.7078, 70.2418) (9.1776, 71.2557) (8.6474, 72.2713) knots 0 0 0 0 1 1 1 1
  spline S181 degree 3 poles (8.6474, 72.2713) (8.5778, 72.4049) (8.5083, 72.5385) (8.4367, 72.6761) knots 0 0 0 0 1 1 1 1
  spline S182 degree 3 poles (8.4367, 72.6761) (8.375, 72.7935) (8.3133, 72.9109) (8.2498, 73.0318) knots 0 0 0 0 1 1 1 1
  spline S183 degree 3 poles (8.2498, 73.0318) (8.1049, 73.3303) (8.1049, 73.3303) (8.0017, 73.7156) knots 0 0 0 0 1 1 1 1
  spline S184 degree 3 poles (8.0017, 73.7156) (7.383, 73.4817) (7.383, 73.4817) (6.7518, 73.2431) knots 0 0 0 0 1 1 1 1
  spline S185 degree 3 poles (6.7518, 73.2431) (6.7354, 73.0492) (6.7191, 72.8553) (6.7022, 72.6555) knots 0 0 0 0 1 1 1 1
  spline S186 degree 3 poles (6.7022, 72.6555) (6.4673, 70.0309) (6.0493, 67.375) (4.0118, 65.4886) knots 0 0 0 0 1 1 1 1
  spline S187 degree 3 poles (4.0118, 65.4886) (3.5344, 65.1735) (3.074, 65.0134) (2.505, 64.9472) knots 0 0 0 0 1 1 1 1
  spline S188 degree 3 poles (2.505, 64.9472) (2.0267, 65.0887) (1.8077, 65.224) (1.5478, 65.6538) knots 0 0 0 0 1 1 1 1
  spline S189 degree 3 poles (1.5478, 65.6538) (1.1645, 66.6642) (1.5003, 67.6789) (1.7413, 68.6857) knots 0 0 0 0 1 1 1 1
  spline S190 degree 3 poles (1.7413, 68.6857) (2.7388, 72.8857) (2.9835, 76.7421) (2.129, 80.9695) knots 0 0 0 0 1 1 1 1
  spline S191 degree 3 poles (2.129, 80.9695) (2.0958, 81.1349) (2.0625, 81.3003) (2.0283, 81.4707) knots 0 0 0 0 1 1 1 1
  spline S192 degree 3 poles (2.0283, 81.4707) (1.9621, 81.7967) (1.8945, 82.1224) (1.8252, 82.4478) knots 0 0 0 0 1 1 1 1
  spline S193 degree 3 poles (1.8252, 82.4478) (1.2314, 85.3444) (1.2314, 85.3444) (1.8197, 86.5126) knots 0 0 0 0 1 1 1 1
  spline S194 degree 3 poles (1.8197, 86.5126) (2.2903, 87.008) (2.7832, 87.1137) (3.4549, 87.0884) knots 0 0 0 0 1 1 1 1
  spline S195 degree 3 poles (62.8723, 105.7623) (63.8123, 105.2136) (64.4641, 104.4032) (64.8194, 103.3761) knots 0 0 0 0 1 1 1 1
  spline S196 degree 3 poles (64.8194, 103.3761) (65.0393, 102.4434) (64.9292, 101.2807) (64.7373, 100.343) knots 0 0 0 0 1 1 1 1
  spline S197 degree 3 poles (64.7373, 100.343) (64.833, 100.3269) (64.9287, 100.3109) (65.0273, 100.2943) knots 0 0 0 0 1 1 1 1
  spline S198 degree 3 poles (65.0273, 100.2943) (65.7751, 100.1573) (66.3766, 100.0201) (67.0079, 99.5749) knots 0 0 0 0 1 1 1 1
  spline S199 degree 3 poles (67.0079, 99.5749) (67.1506, 99.4768) (67.2933, 99.3788) (67.4403, 99.2778) knots 0 0 0 0 1 1 1 1
  spline S200 degree 3 poles (67.4403, 99.2778) (68.4473, 98.4209) (69.0645, 97.166) (69.1903, 95.865) knots 0 0 0 0 1 1 1 1
  spline S201 degree 3 poles (69.1903, 95.865) (69.2075, 94.4689) (68.2873, 93.0873) (67.3595, 92.0982) knots 0 0 0 0 1 1 1 1
  spline S202 degree 3 poles (67.3595, 92.0982) (66.8176, 91.5893) (66.247, 91.1167) (65.6648, 90.655) knots 0 0 0 0 1 1 1 1
  spline S203 degree 3 poles (65.6648, 90.655) (65.4967, 90.5217) (65.331, 90.3854) (65.1662, 90.248) knots 0 0 0 0 1 1 1 1
  spline S204 degree 3 poles (65.1662, 90.248) (64.6092, 89.8249) (63.993, 89.6418) (63.3281, 89.4522) knots 0 0 0 0 1 1 1 1
  spline S205 degree 3 poles (63.3281, 89.4522) (63.2372, 89.4259) (63.1463, 89.3996) (63.0526, 89.3725) knots 0 0 0 0 1 1 1 1
  spline S206 degree 3 poles (63.0526, 89.3725) (62.7916, 89.3052) (62.7916, 89.3052) (62.3439, 89.2401) knots 0 0 0 0 1 1 1 1
  spline S207 degree 3 poles (62.3439, 89.2401) (61.9981, 89.5441) (61.8594, 89.7425) (61.6426, 90.1378) knots 0 0 0 0 1 1 1 1
  spline S208 degree 3 poles (61.6426, 90.1378) (61.5719, 90.2643) (61.5011, 90.3909) (61.4283, 90.5212) knots 0 0 0 0 1 1 1 1
  spline S209 degree 3 poles (61.4283, 90.5212) (61.3491, 90.6634) (61.2699, 90.8057) (61.1883, 90.9523) knots 0 0 0 0 1 1 1 1
  spline S210 degree 3 poles (61.1883, 90.9523) (60.4543, 92.2554) (59.6823, 93.5307) (58.8855, 94.7965) knots 0 0 0 0 1 1 1 1
  spline S211 degree 3 poles (58.8855, 94.7965) (58.7937, 94.9426) (58.7019, 95.0887) (58.6073, 95.2392) knots 0 0 0 0 1 1 1 1
  spline S212 degree 3 poles (58.6073, 95.2392) (58.1408, 95.9809) (57.6722, 96.7212) (57.2012, 97.46) knots 0 0 0 0 1 1 1 1
  spline S213 degree 3 poles (57.2012, 97.46) (57.0254, 97.7387) (56.8496, 98.0175) (56.6739, 98.2964) knots 0 0 0 0 1 1 1 1
  spline S214 degree 3 poles (56.6739, 98.2964) (56.5923, 98.4229) (56.5107, 98.5495) (56.4266, 98.6799) knots 0 0 0 0 1 1 1 1
  spline S215 degree 3 poles (56.4266, 98.6799) (55.9583, 99.427) (55.592, 100.1425) (55.4694, 101.0256) knots 0 0 0 0 1 1 1 1
  spline S216 degree 3 poles (55.4694, 101.0256) (55.8662, 102.6522) (58.2889, 104.2956) (59.6555, 105.1362) knots 0 0 0 0 1 1 1 1
  spline S217 degree 3 poles (59.6555, 105.1362) (60.6471, 105.7071) (61.7485, 106.1192) (62.8723, 105.7623) knots 0 0 0 0 1 1 1 1
  spline S218 degree 3 poles (-4.3854, 87.6804) (-3.5049, 87.3156) (-2.914, 86.74) (-2.4277, 85.9251) knots 0 0 0 0 1 1 1 1
  spline S219 degree 3 poles (-2.4277, 85.9251) (-2.0978, 85.1213) (-1.8762, 84.351) (-2.1936, 83.5101) knots 0 0 0 0 1 1 1 1
  spline S220 degree 3 poles (-2.1936, 83.5101) (-2.4262, 83.0534) (-2.6, 82.9888) (-3.0867, 82.7976) knots 0 0 0 0 1 1 1 1
  spline S221 degree 3 poles (-3.0867, 82.7976) (-3.9689, 82.5994) (-4.6124, 83.061) (-5.354, 83.4892) knots 0 0 0 0 1 1 1 1
  spline S222 degree 3 poles (-5.354, 83.4892) (-5.8603, 83.5196) (-6.1948, 83.446) (-6.6727, 83.2735) knots 0 0 0 0 1 1 1 1
  spline S223 degree 3 poles (-6.6727, 83.2735) (-8.2016, 81.8954) (-8.3683, 79.4894) (-8.4896, 77.5645) knots 0 0 0 0 1 1 1 1
  spline S224 degree 3 poles (-8.4896, 77.5645) (-8.6179, 75.0795) (-8.5889, 72.1816) (-6.9995, 70.109) knots 0 0 0 0 1 1 1 1
  spline S225 degree 3 poles (-6.9995, 70.109) (-6.4165, 69.4795) (-5.8107, 69.1952) (-4.9514, 69.1436) knots 0 0 0 0 1 1 1 1
  spline S226 degree 3 poles (-4.9514, 69.1436) (-4.4929, 69.2397) (-4.0372, 69.3449) (-3.5812, 69.4522) knots 0 0 0 0 1 1 1 1
  spline S227 degree 3 poles (-3.5812, 69.4522) (-3.0492, 69.5037) (-2.7964, 69.4233) (-2.3391, 69.1553) knots 0 0 0 0 1 1 1 1
  spline S228 degree 3 poles (-2.3391, 69.1553) (-1.9688, 68.5944) (-1.7451, 68.0204) (-1.8415, 67.3401) knots 0 0 0 0 1 1 1 1
  spline S229 degree 3 poles (-1.8415, 67.3401) (-2.1526, 66.3969) (-2.8124, 65.7695) (-3.6277, 65.2311) knots 0 0 0 0 1 1 1 1
  spline S230 degree 3 poles (-3.6277, 65.2311) (-5.0192, 64.596) (-6.5671, 64.7508) (-7.9922, 65.2069) knots 0 0 0 0 1 1 1 1
  spline S231 degree 3 poles (-7.9922, 65.2069) (-9.8133, 65.9349) (-10.9, 67.5757) (-11.6735, 69.3042) knots 0 0 0 0 1 1 1 1
  spline S232 degree 3 poles (-11.6735, 69.3042) (-13.2889, 73.2475) (-13.5501, 77.612) (-12.4521, 81.7249) knots 0 0 0 0 1 1 1 1
  spline S233 degree 3 poles (-12.4521, 81.7249) (-12.4281, 81.8161) (-12.4041, 81.9072) (-12.3794, 82.0012) knots 0 0 0 0 1 1 1 1
  spline S234 degree 3 poles (-12.3794, 82.0012) (-11.8408, 83.988) (-10.9642, 85.7449) (-9.2546, 86.9693) knots 0 0 0 0 1 1 1 1
  spline S235 degree 3 poles (-9.2546, 86.9693) (-7.7966, 87.8051) (-5.9908, 88.2088) (-4.3854, 87.6804) knots 0 0 0 0 1 1 1 1
  spline S236 degree 3 poles (51.7978, 98.803) (53.0736, 98.4533) (53.9973, 97.4017) (54.6398, 96.2915) knots 0 0 0 0 1 1 1 1
  spline S237 degree 3 poles (54.6398, 96.2915) (54.7715, 96.0448) (54.9006, 95.7967) (55.0274, 95.5474) knots 0 0 0 0 1 1 1 1
  spline S238 degree 3 poles (55.0274, 95.5474) (55.097, 95.413) (55.1667, 95.2787) (55.2384, 95.1402) knots 0 0 0 0 1 1 1 1
  spline S239 degree 3 poles (55.2384, 95.1402) (58.1865, 89.3546) (58.1865, 89.3546) (57.9109, 86.2628) knots 0 0 0 0 1 1 1 1
  spline S240 degree 3 poles (57.9109, 86.2628) (57.9017, 86.1429) (57.8925, 86.023) (57.883, 85.8994) knots 0 0 0 0 1 1 1 1
  spline S241 degree 3 poles (57.883, 85.8994) (57.7542, 84.7714) (57.3255, 83.8312) (56.4564, 83.092) knots 0 0 0 0 1 1 1 1
  spline S242 degree 3 poles (56.4564, 83.092) (55.9917, 82.7739) (55.4926, 82.6427) (54.9504, 82.5101) knots 0 0 0 0 1 1 1 1
  spline S243 degree 3 poles (54.9504, 82.5101) (54.7801, 82.4669) (54.7801, 82.4669) (54.6063, 82.4229) knots 0 0 0 0 1 1 1 1
  spline S244 degree 3 poles (54.6063, 82.4229) (52.9272, 82.0273) (51.6233, 82.3586) (50.1687, 83.242) knots 0 0 0 0 1 1 1 1
  spline S245 degree 3 poles (50.1687, 83.242) (48.6083, 84.3441) (47.7412, 85.9458) (46.7895, 87.5599) knots 0 0 0 0 1 1 1 1
  spline S246 degree 3 poles (46.7895, 87.5599) (46.5586, 87.9512) (46.3257, 88.3413) (46.0925, 88.7312) knots 0 0 0 0 1 1 1 1
  spline S247 degree 3 poles (46.0925, 88.7312) (43.4716, 93.1281) (43.4716, 93.1281) (43.6287, 94.2708) knots 0 0 0 0 1 1 1 1
  spline S248 degree 3 poles (43.6287, 94.2708) (43.7356, 94.6135) (43.8492, 94.854) (44.1196, 95.0938) knots 0 0 0 0 1 1 1 1
  spline S249 degree 3 poles (44.1196, 95.0938) (44.9932, 95.4063) (44.9932, 95.4063) (45.5518, 95.2711) knots 0 0 0 0 1 1 1 1
  spline S250 degree 3 poles (45.5518, 95.2711) (46.5195, 94.6423) (47.0156, 93.6682) (47.5526, 92.6804) knots 0 0 0 0 1 1 1 1
  spline S251 degree 3 poles (47.5526, 92.6804) (47.6302, 92.5403) (47.7078, 92.4002) (47.7877, 92.2558) knots 0 0 0 0 1 1 1 1
  spline S252 degree 3 poles (47.7877, 92.2558) (48.0348, 91.8093) (48.2805, 91.3621) (48.5258, 90.9146) knots 0 0 0 0 1 1 1 1
  spline S253 degree 3 poles (48.5258, 90.9146) (50.075, 87.8445) (50.075, 87.8445) (52.1567, 85.134) knots 0 0 0 0 1 1 1 1
  spline S254 degree 3 poles (52.1567, 85.134) (52.8596, 84.9395) (53.538, 85.1409) (54.1749, 85.4683) knots 0 0 0 0 1 1 1 1
  spline S255 degree 3 poles (54.1749, 85.4683) (54.5057, 85.9706) (54.4847, 86.6066) (54.4022, 87.1852) knots 0 0 0 0 1 1 1 1
  spline S256 degree 3 poles (54.4022, 87.1852) (54.3203, 87.5614) (54.2246, 87.9307) (54.1212, 88.3015) knots 0 0 0 0 1 1 1 1
  spline S257 degree 3 poles (54.1212, 88.3015) (54.0643, 88.5087) (54.0643, 88.5087) (54.0062, 88.7201) knots 0 0 0 0 1 1 1 1
  spline S258 degree 3 poles (54.0062, 88.7201) (53.3508, 90.9917) (52.4083, 93.1711) (51.1935, 95.1982) knots 0 0 0 0 1 1 1 1
  spline S259 degree 3 poles (51.1935, 95.1982) (50.7008, 96.0267) (50.3882, 96.7187) (50.4881, 97.6864) knots 0 0 0 0 1 1 1 1
  spline S260 degree 3 poles (50.4881, 97.6864) (50.7483, 98.47) (50.9162, 98.7151) (51.7978, 98.803) knots 0 0 0 0 1 1 1 1
  spline S261 degree 3 poles (28.8559, 88.0358) (29.1288, 87.9546) (29.1288, 87.9546) (29.4053, 87.8475) knots 0 0 0 0 1 1 1 1
  spline S262 degree 3 poles (29.4053, 87.8475) (29.5103, 87.8087) (29.6153, 87.7699) (29.7234, 87.73) knots 0 0 0 0 1 1 1 1
  spline S263 degree 3 poles (29.7234, 87.73) (30.6299, 87.3429) (31.3736, 86.7471) (31.786, 85.8318) knots 0 0 0 0 1 1 1 1
  spline S264 degree 3 poles (31.786, 85.8318) (31.9261, 85.3683) (31.9896, 84.9594) (31.8161, 84.5015) knots 0 0 0 0 1 1 1 1
  spline S265 degree 3 poles (31.8161, 84.5015) (31.502, 84.223) (31.2342, 84.1743) (30.823, 84.0978) knots 0 0 0 0 1 1 1 1
  spline S266 degree 3 poles (30.823, 84.0978) (30.4342, 84.1743) (30.4342, 84.1743) (30.0375, 84.3003) knots 0 0 0 0 1 1 1 1
  spline S267 degree 3 poles (30.0375, 84.3003) (29.2905, 84.4967) (28.7399, 84.5594) (28.0479, 84.1801) knots 0 0 0 0 1 1 1 1
  spline S268 degree 3 poles (28.0479, 84.1801) (27.3807, 83.6762) (27.2089, 83.0309) (27.0608, 82.2353) knots 0 0 0 0 1 1 1 1
  spline S269 degree 3 poles (27.0608, 82.2353) (26.9626, 81.2109) (27.0965, 80.3544) (27.3669, 79.3691) knots 0 0 0 0 1 1 1 1
  spline S270 degree 3 poles (27.3669, 79.3691) (27.4009, 79.2447) (27.4349, 79.1203) (27.4699, 78.9921) knots 0 0 0 0 1 1 1 1
  spline S271 degree 3 poles (27.4699, 78.9921) (28.0509, 76.9565) (29.1768, 74.8564) (31.0637, 73.7518) knots 0 0 0 0 1 1 1 1
  spline S272 degree 3 poles (31.0637, 73.7518) (31.7564, 73.4142) (32.2396, 73.4207) (32.979, 73.6214) knots 0 0 0 0 1 1 1 1
  spline S273 degree 3 poles (32.979, 73.6214) (33.3893, 73.7819) (33.7243, 74.0014) (34.091, 74.2452) knots 0 0 0 0 1 1 1 1
  spline S274 degree 3 poles (34.091, 74.2452) (34.7264, 74.6609) (35.1495, 74.8825) (35.913, 74.8625) knots 0 0 0 0 1 1 1 1
  spline S275 degree 3 poles (35.913, 74.8625) (36.4167, 74.5693) (36.5455, 74.265) (36.6943, 73.7125) knots 0 0 0 0 1 1 1 1
  spline S276 degree 3 poles (36.6943, 73.7125) (36.8548, 73.0352) (36.876, 72.6345) (36.5417, 72.0026) knots 0 0 0 0 1 1 1 1
  spline S277 degree 3 poles (36.5417, 72.0026) (36.5013, 71.9215) (36.4609, 71.8404) (36.4193, 71.7568) knots 0 0 0 0 1 1 1 1
  spline S278 degree 3 poles (36.4193, 71.7568) (35.711, 70.523) (34.4004, 69.9989) (33.0902, 69.6324) knots 0 0 0 0 1 1 1 1
  spline S279 degree 3 poles (33.0902, 69.6324) (32.1761, 69.3982) (31.3786, 69.2762) (30.455, 69.5457) knots 0 0 0 0 1 1 1 1
  spline S280 degree 3 poles (30.455, 69.5457) (30.3523, 69.575) (30.2495, 69.6042) (30.1436, 69.6344) knots 0 0 0 0 1 1 1 1
  spline S281 degree 3 poles (30.1436, 69.6344) (27.8537, 70.4248) (26.5565, 72.4937) (25.5328, 74.5588) knots 0 0 0 0 1 1 1 1
  spline S282 degree 3 poles (25.5328, 74.5588) (25.2503, 75.2206) (25.0164, 75.8808) (24.8224, 76.5741) knots 0 0 0 0 1 1 1 1
  spline S283 degree 3 poles (24.8224, 76.5741) (24.7957, 76.6687) (24.7689, 76.7634) (24.7414, 76.8609) knots 0 0 0 0 1 1 1 1
  spline S284 degree 3 poles (24.7414, 76.8609) (23.9313, 79.7605) (23.0582, 82.9787) (24.6205, 85.8239) knots 0 0 0 0 1 1 1 1
  spline S285 degree 3 poles (24.6205, 85.8239) (25.5895, 87.1683) (27.0919, 88.3422) (28.8559, 88.0358) knots 0 0 0 0 1 1 1 1
  spline S286 degree 3 poles (35.271, 91.0968) (35.9056, 91.0279) (36.2546, 90.7872) (36.7167, 90.3571) knots 0 0 0 0 1 1 1 1
  spline S287 degree 3 poles (36.7167, 90.3571) (38.7859, 87.6056) (39.8668, 84.1739) (40.9285, 80.9374) knots 0 0 0 0 1 1 1 1
  spline S288 degree 3 poles (40.9285, 80.9374) (40.976, 80.7927) (40.976, 80.7927) (41.0245, 80.6452) knots 0 0 0 0 1 1 1 1
  spline S289 degree 3 poles (41.0245, 80.6452) (41.0845, 80.4618) (41.144, 80.2782) (41.203, 80.0945) knots 0 0 0 0 1 1 1 1
  spline S290 degree 3 poles (41.203, 80.0945) (41.4245, 79.415) (41.7016, 78.7821) (42.05, 78.1587) knots 0 0 0 0 1 1 1 1
  spline S291 degree 3 poles (42.05, 78.1587) (43.3628, 78.4342) (44.5032, 78.8064) (45.6724, 79.4734) knots 0 0 0 0 1 1 1 1
  spline S292 degree 3 poles (45.6724, 79.4734) (46.8703, 80.155) (48.0255, 80.7884) (49.4302, 80.4115) knots 0 0 0 0 1 1 1 1
  spline S293 degree 3 poles (49.4302, 80.4115) (49.7165, 80.0886) (49.7707, 79.8458) (49.8339, 79.4185) knots 0 0 0 0 1 1 1 1
  spline S294 degree 3 poles (49.8339, 79.4185) (49.5791, 78.3853) (48.7694, 77.9162) (47.9007, 77.3863) knots 0 0 0 0 1 1 1 1
  spline S295 degree 3 poles (47.9007, 77.3863) (46.9562, 76.8279) (45.9936, 76.3046) (45.0248, 75.7898) knots 0 0 0 0 1 1 1 1
  spline S296 degree 3 poles (45.0248, 75.7898) (44.9318, 75.7396) (44.8388, 75.6894) (44.743, 75.6376) knots 0 0 0 0 1 1 1 1
  spline S297 degree 3 poles (44.743, 75.6376) (43.781, 75.1223) (42.8167, 74.7496) (41.7675, 74.461) knots 0 0 0 0 1 1 1 1
  spline S298 degree 3 poles (41.7675, 74.461) (41.6635, 74.4324) (41.5595, 74.4037) (41.4524, 74.3742) knots 0 0 0 0 1 1 1 1
  spline S299 degree 3 poles (41.4524, 74.3742) (40.9456, 74.2452) (40.5505, 74.1474) (40.0505, 74.3193) knots 0 0 0 0 1 1 1 1
  spline S300 degree 3 poles (40.0505, 74.3193) (39.8885, 74.5225) (39.8885, 74.5225) (39.7642, 74.7881) knots 0 0 0 0 1 1 1 1
  spline S301 degree 3 poles (39.7642, 74.7881) (39.7175, 74.8869) (39.6708, 74.9857) (39.6226, 75.0874) knots 0 0 0 0 1 1 1 1
  spline S302 degree 3 poles (39.6226, 75.0874) (39.3875, 75.6278) (39.1636, 76.1713) (38.9485, 76.72) knots 0 0 0 0 1 1 1 1
  spline S303 degree 3 poles (38.9485, 76.72) (38.8463, 76.9776) (38.744, 77.2352) (38.6418, 77.4928) knots 0 0 0 0 1 1 1 1
  spline S304 degree 3 poles (38.6418, 77.4928) (38.589, 77.6265) (38.5361, 77.7603) (38.4817, 77.8981) knots 0 0 0 0 1 1 1 1
  spline S305 degree 3 poles (38.4817, 77.8981) (37.5916, 80.15) (36.6822, 82.3915) (35.7178, 84.6127) knots 0 0 0 0 1 1 1 1
  spline S306 degree 3 poles (35.7178, 84.6127) (33.9095, 88.7826) (33.9095, 88.7826) (34.2941, 90.0489) knots 0 0 0 0 1 1 1 1
  spline S307 degree 3 poles (34.2941, 90.0489) (34.5273, 90.5928) (34.697, 90.9031) (35.271, 91.0968) knots 0 0 0 0 1 1 1 1
  spline S308 degree 3 poles (65.322, 97.5831) (65.9067, 97.3047) (66.3169, 97.0475) (66.6048, 96.4557) knots 0 0 0 0 1 1 1 1
  spline S309 degree 3 poles (66.6048, 96.4557) (66.8023, 95.8848) (66.7295, 95.4286) (66.474, 94.8893) knots 0 0 0 0 1 1 1 1
  spline S310 degree 3 poles (66.474, 94.8893) (65.8194, 93.6997) (64.6944, 92.9708) (63.6165, 92.1965) knots 0 0 0 0 1 1 1 1
  spline S311 degree 3 poles (63.6165, 92.1965) (63.2564, 92.513) (63.103, 92.7491) (62.8745, 93.164) knots 0 0 0 0 1 1 1 1
  spline S312 degree 3 poles (62.8745, 93.164) (62.8039, 93.2915) (62.7333, 93.4191) (62.6606, 93.5505) knots 0 0 0 0 1 1 1 1
  spline S313 degree 3 poles (62.6606, 93.5505) (62.5878, 93.6839) (62.515, 93.8172) (62.44, 93.9546) knots 0 0 0 0 1 1 1 1
  spline S314 degree 3 poles (62.44, 93.9546) (62.366, 94.0882) (62.2921, 94.2218) (62.2159, 94.3594) knots 0 0 0 0 1 1 1 1